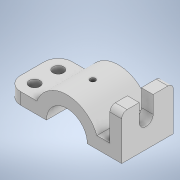
# Autodesk Inventor part: 2.7
Saved by Autodesk Inventor 2022 (Build 260153000, 153)
## iProperties
Created: 2023-04-17
Part Number: 2.7
Material: Genérico
Document SubType Name: Modeling
Designer: jpjoa
Density: 1 g/cm^3
Appearance: Padrão
Author: jpjoa
Autodesk Inventor part; units mm, degrees
ref_plane "YZ Plane" through (0, 0, 0) normal (1, 0, 0) x (0, 1, 0)
ref_plane "XZ Plane" through (0, 0, 0) normal (0, 1, 0) x (-1, 0, 0)
ref_plane "XY Plane" through (0, 0, 0) normal (0, 0, 1) x (1, 0, 0)
sketch "Esboço1" plane through (0, 0, 0) normal (0, 0, 1) x (1, 0, 0)
  arc A0 (75, 0) -> (37, 0) centre (56, 0) ccw
  line L0 (75, 0) -> (107, 0)
  line L1 (0, 0) -> (37, 0)
  line L2 (107, 0) -> (107, 41)
  line L3 (0, 11) -> (28.0894, 11)
  arc A1 (83.9106, 11) -> (28.0894, 11) centre (56, 0) ccw
  line L4 (83.9106, 11) -> (96, 11)
  line L5 (96, 11) -> (96, 41)
  line L6 (0, 11) -> (0, 0)
  line L7 (96, 41) -> (107, 41)
  dimension "d0" = 38
  dimension "d5" = 41
  dimension "d6" = 51
  dimension "d7" = 107
  dimension "d8" = 11
  constraints: 16 end point, 4 point on circle, 2 centre point, 2 coincident, 2 horizontal, 2 horizontal alignment, 2 vertical, 1 perpendicular, 3 other
  measures "d0" diameter of A0
  measures "d5" distance of L0.end L2.end
  measures "d6" distance from line of L2 A0.centre
  measures "d7" distance of L0.end point (0, 0)
  measures "d8" radial gap between concentric circles of A0 A1
extrude "Extrusão1" add sketch "Esboço1" along normal blind 48
sketch "Esboço2" plane through (0, 11, 0) normal (0, 1, 0) x (1, 0, 0)
  circle A0 centre (13, -35) radius 5
  circle A1 centre (13, -13) radius 5
  line L0 (28.0894, -48) -> (0, -48) projected
  line L1 (0, 0) -> (0, -48) projected
  circle A2 centre (55.9996, -24) radius 2.5
  line L2 (28.0894, 0) -> (83.9106, 0) projected
  line L3 (28.0894, -48) -> (83.9106, -48) projected
  line L4 (83.9106, 0) -> (83.9106, -48) projected
  line L5 (28.0894, 0) -> (28.0894, -48) projected
  dimension "d11" = 10
  dimension "d12" = 10
  dimension "d13" = 22
  dimension "d14" = 13
  dimension "d15" = 13
  dimension "d16" = 5
  dimension "d17" = 24
  dimension "d19" = 27.911
  constraints: 3 centre point, 1 vertical alignment
  measures "d11" diameter of A0
  measures "d12" diameter of A1
  measures "d13" distance of A1.centre A0.centre
  measures "d14" distance from line of L0 A0.centre
  measures "d15" distance from line of L1 A1.centre
  measures "d16" diameter of A2
  measures "d17" distance from line of L2 A2.centre
  measures "d19" distance from line of L4 A2.centre
extrude "Extrusão2" cut sketch "Esboço2" along normal through all both and the other way through all contours A0 | A1 | A2
sketch "Esboço3" plane through (107, 0, 0) normal (1, 0, 0) x (0, 0, -1)
  circle A0 centre (-25.2522, 25) radius 6.5
  line L0 (0, 0) -> (-48, 0) projected
  line L1 (-18.7522, 41) -> (-18.7522, 25)
  line L2 (-31.7522, 41) -> (-31.7522, 25)
  line L3 (0, 41) -> (-48, 41) projected
  line L4 (-31.7522, 41) -> (-18.7522, 41)
  dimension "d23" = 13
  dimension "d24" = 25
  constraints: 6 end point, 2 point on circle, 2 point on line, 2 tangent, 2 vertical, 1 centre point
  measures "d23" diameter of A0
  measures "d24" distance from line of L0 A0.centre
extrude "Extrusão3" cut sketch "Esboço3" against normal up to surface (11 mm away)
fillet "Arredondamento1" radius 13 2 edges at (0, 5.5, 0) (0, 5.5, 48)
fillet "Arredondamento2" radius 5 2 edges at (101.5, 41, 0) (101.5, 41, 48)
